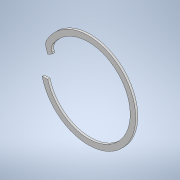
# Autodesk Inventor part: 68. Кольцо стопорное подшипника
Saved by Autodesk Inventor 2021 (Build 250183000, 183)
## iProperties
Created: 2021-03-20
Part Number: 68. Кольцо стопорное подшипника
Material: Типовые
Document SubType Name: Modeling
Designer: Данил
Density: 1 g/cm^3
Appearance: По умолчанию
Author: Данил
Autodesk Inventor part; units mm, degrees
ref_plane "YZ Plane" through (0, 0, 0) normal (1, 0, 0) x (0, 1, 0)
ref_plane "XZ Plane" through (0, 0, 0) normal (0, 1, 0) x (-1, 0, 0)
ref_plane "XY Plane" through (0, 0, 0) normal (0, 0, 1) x (1, 0, 0)
sketch "Эскиз1" plane through (0, 0, 0) normal (0, 0, 1) x (1, 0, 0)
  arc A0 (-21.1675, -5) -> (-19.1116, 10.383) centre (0, 0) ccw
  arc A1 (-18.5893, -5) -> (-16.246, 10.3262) centre (0, 0) ccw
  line L0 (-18.5893, 5) -> (-18.5893, -5) construction
  line L1 (-19.3556, 7.1054) -> (-18.5893, 5)
  line L2 (-18.5893, 5) -> (-16.4242, 6.25)
  line L3 (-16.4242, 6.25) -> (-16.629, 6.8124)
  line L4 (-18.5893, 0) -> (0, 0) construction
  arc A2 (-19.1116, 10.383) -> (-19.3556, 7.1054) centre (-15.5969, 8.4735) ccw
  arc A3 (-16.246, 10.3262) -> (-16.629, 6.8124) centre (-12.8702, 8.1805) ccw
  line L5 (-21.1675, -5) -> (-18.5893, -5)
  point P0 (-19.9352, 8.6978)
  point P1 (-17.2553, 8.5333)
  dimension "d0" = 21.75
  dimension "d1" = 2.5
  dimension "d4" = 10
  dimension "d6" = 30
  dimension "d7" = 100
  dimension "d8" = 2.5
  dimension "d9" = 4
  constraints: 12 end point, 10 point on circle, 4 centre point, 4 tangent, 2 coincident, 2 horizontal, 2 horizontal alignment, 2 point on line, 1 equal radius, 1 midpoint, 1 parallel, 1 vertical
  measures "d0" radius of A0
  measures "d1" radial gap between concentric circles of A0 A1
  measures "d4" distance of L0.start L0.end
  measures "d6" angle of L4 L2
  measures "d7" angle of L2 L3
  measures "d8" distance of L0.start L2.end
  measures "d9" radius of A2
extrude "Выдавливание1" add sketch "Эскиз1" along normal mid plane 1
